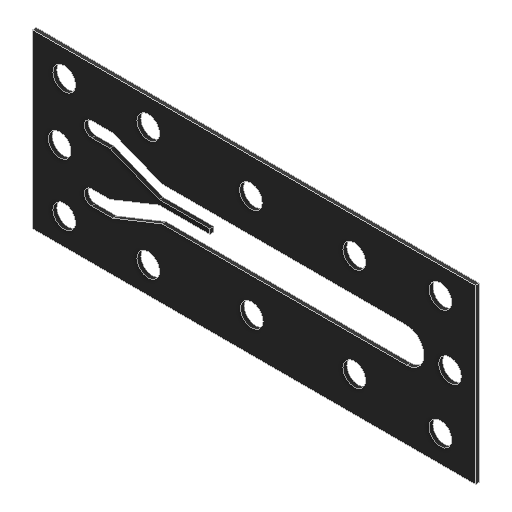
# Autodesk Inventor part: borracha vedação
Saved by Autodesk Inventor 2025 (Build 290162000, 162)
## iProperties
Created: 2024-12-11
Part Number: borracha vedação
Material: Genérico
Document SubType Name: Modeling
Designer: November
Density: 1 g/cm^3
Appearance: Borracha - Preta
Author: November
Autodesk Inventor part; units mm, degrees
ref_plane "YZ Plane" through (0, 0, 0) normal (1, 0, 0) x (0, 1, 0)
ref_plane "XZ Plane" through (0, 0, 0) normal (0, 1, 0) x (-1, 0, 0)
ref_plane "XY Plane" through (0, 0, 0) normal (0, 0, 1) x (1, 0, 0)
sketch "Esboço1" plane through (0, 0, 0) normal (0, 0, 1) x (1, 0, 0)
  line L0 (-5.298, 38.5267) -> (-95.2722, 38.5267)
  line L1 (-95.2722, 38.5267) -> (-95.2722, 3.5267)
  line L2 (-95.2722, 3.5267) -> (-5.298, 3.5267)
  line L3 (-5.298, 3.5267) -> (-5.298, 38.5267)
  line L4 (-78.9833, 28.5267) -> (-68.9833, 24.5267)
  line L5 (-68.9833, 24.5267) -> (-19.298, 24.5267)
  arc A0 (-19.298, 17.5267) -> (-19.298, 24.5267) centre (-19.298, 21.0267) ccw
  line L6 (-19.298, 17.5267) -> (-68.9833, 17.5267)
  line L7 (-68.9833, 17.5267) -> (-78.9833, 13.5267)
  line L8 (-78.9833, 13.5267) -> (-83.2722, 13.5267)
  arc A1 (-83.2722, 16.5267) -> (-83.2722, 13.5267) centre (-83.2722, 15.0267) ccw
  line L9 (-83.2722, 16.5267) -> (-79.561, 16.5267)
  line L10 (-79.561, 16.5267) -> (-69.561, 20.5267)
  line L11 (-69.561, 20.5267) -> (-59.2722, 20.5267)
  line L12 (-59.2722, 20.5267) -> (-59.2722, 21.5267)
  line L13 (-59.2722, 21.5267) -> (-69.561, 21.5267)
  line L14 (-69.561, 21.5267) -> (-79.561, 25.5267)
  line L15 (-79.561, 25.5267) -> (-83.2722, 25.5267)
  arc A2 (-83.2722, 28.5267) -> (-83.2722, 25.5267) centre (-83.2722, 27.0267) ccw
  line L16 (-83.2722, 28.5267) -> (-78.9833, 28.5267)
  circle A3 centre (-29.9293, 31.4267) radius 2.3
  circle A4 centre (-50.9293, 31.4267) radius 2.3
  circle A5 centre (-29.9293, 10.6267) radius 2.3
  circle A6 centre (-71.7596, 8.9271) radius 2.3
  circle A7 centre (-50.7596, 10.6267) radius 2.3
  circle A8 centre (-10.4983, 21.0267) radius 2.3
  circle A9 centre (-89.7596, 21.0267) radius 2.3
  circle A10 centre (-71.7596, 33.1263) radius 2.3
  circle A11 centre (-88.8351, 33.1263) radius 2.3
  circle A12 centre (-88.8351, 8.9271) radius 2.3
  circle A13 centre (-12.4442, 33.1263) radius 2.3
  circle A14 centre (-12.4515, 8.9271) radius 2.3
  point P0 (0, 0)
  constraints: 34 end point, 15 centre point, 6 point on circle
extrude "Extrusão1" add sketch "Esboço1" along normal blind 0.8
